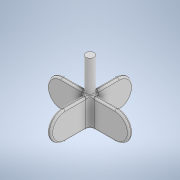
# Autodesk Inventor part: torniquete
Saved by Autodesk Inventor 2022 (Build 260153000, 153)
## iProperties
Created: 2022-11-08
Part Number: torniquete
Material: Generic
Document SubType Name: Modeling
Designer: 3.6b
Density: 1 g/cm^3
Appearance: Default
Author: 3.6b
Autodesk Inventor part; units mm, degrees
ref_plane "YZ Plane" through (0, 0, 0) normal (1, 0, 0) x (0, 1, 0)
ref_plane "XZ Plane" through (0, 0, 0) normal (0, 1, 0) x (-1, 0, 0)
ref_plane "XY Plane" through (0, 0, 0) normal (0, 0, 1) x (1, 0, 0)
sketch "Sketch1" plane through (0, 0, 0) normal (0, 1, 0) x (-1, 0, 0)
  line L0 (33, 2.5) -> (33, -2.5)
  line L1 (-33, -2.5) -> (-33, 2.5)
  line L2 (-33, 2.5) -> (33, -2.5) construction
  line L3 (33, 2.5) -> (-33, -2.5) construction
  line L4 (2.5, 33) -> (-2.5, 33)
  line L5 (-2.5, -33) -> (2.5, -33)
  line L6 (2.5, 33) -> (-2.5, -33) construction
  line L7 (-2.5, 33) -> (2.5, -33) construction
  line L8 (-2.5, 33) -> (-2.5, 2.5)
  line L9 (-2.5, -2.5) -> (-2.5, -33)
  line L10 (2.5, 2.5) -> (2.5, 33)
  line L11 (2.5, -33) -> (2.5, -2.5)
  line L12 (33, -2.5) -> (2.5, -2.5)
  line L13 (-2.5, -2.5) -> (-33, -2.5)
  line L14 (2.5, 2.5) -> (33, 2.5)
  line L15 (-33, 2.5) -> (-2.5, 2.5)
  point P0 (0, 0)
  dimension "d0" = 66
  dimension "d1" = 5
  dimension "d2" = 5
  dimension "d3" = 66
  constraints: 32 end point, 10 parallel, 4 midpoint, 4 perpendicular, 3 horizontal
  measures "d0" distance of L0.end L1.start
  measures "d1" distance of L0.start L0.end
  measures "d2" distance of L5.end L5.start
  measures "d3" distance of L5.start L4.end
extrude "Extrusion1" add sketch "Sketch1" along normal blind 34
sketch "Sketch3" plane through (2.5, 0, 2.5) normal (0, 0, 1) x (1, 0, 0)
  line L0 (30.5, 0) -> (30.5, 34) projected
  line L1 (0, 0) -> (30.5, 0) projected
  arc A0 (30.5, 0) -> (30.5, 34) centre (30.5, 17) ccw
  line L2 (-35.5, 0) -> (-35.5, 34) projected
  arc A1 (-35.5, 34) -> (-35.5, 0) centre (-35.5, 17) ccw
  point P0 (-2.5, 0)
  constraints: 4 end point, 4 point on circle, 2 centre point, 2 midpoint
extrude "Extrusion2" add sketch "Sketch3" against normal blind 5
sketch "Sketch4" plane through (-2.5, 0, -33) normal (-1, 0, 0) x (0, 0, 1)
  line L0 (0, 0) -> (0, 34) projected
  line L1 (0, 34) -> (30.5, 34) projected
  arc A0 (0, 34) -> (0, 0) centre (0, 17) ccw
  line L2 (66, 0) -> (66, 34) projected
  arc A1 (66, 0) -> (66, 34) centre (66, 17) ccw
  point P0 (33, 0)
  constraints: 4 end point, 4 point on circle, 2 centre point, 2 midpoint
extrude "Extrusion3" add sketch "Sketch4" against normal blind 5
sketch "Sketch5" plane through (0, 34, 0) normal (0, 1, 0) x (1, 0, 0)
  circle A0 centre (0, 0) radius 5
  dimension "d10" = 10
  constraints: 1 centre point, 1 coincident
  measures "d10" diameter of A0
extrude "Extrusion4" add sketch "Sketch5" along normal blind 40
fillet "Fillet1" radius 5 1 edges at (-2.5, 17, 2.5)
fillet "Fillet2" radius 5 3 edges at (2.5, 17, 2.5) (2.5, 17, -2.5) (-2.5, 17, -2.5)
fillet "Fillet3" radius 2 1 edges at (-5, 34, 0)
fillet "Fillet4" radius 2 40 edges at (3.9668, 34.5653, 3.9622) (2.5254, 34, 6.9968) (2.5, 34, 20.25) (2.5, 17, 50) (2.5, 0, 20.25) (3.9645, 0, 3.9645) (20.25, 0, 2.5) (50, 17, 2.5) (20.25, 34, 2.5) (6.9968, 34, 2.5254) (6.9968, 34, -2.5254) (20.25, 34, -2.5) (50, 17, -2.5) (20.25, 0, -2.5) (3.9645, 0, -3.9645) (2.5, 0, -20.25) (2.5, 17, -50) (2.5, 34, -20.25) (2.5254, 34, -6.9968) (3.9622, 34.5653, -3.9668) (-2.5254, 34, -6.9968) (-2.5, 34, -20.25) (-2.5, 17, -50) (-2.5, 0, -20.25) (-3.9645, 0, -3.9645) (-20.25, 0, -2.5) (-50, 17, -2.5) (-20.25, 34, -2.5) (-6.9968, 34, -2.5254) (-3.9668, 34.5653, -3.9622) (-6.9968, 34, 2.5254) (-20.25, 34, 2.5) (-50, 17, 2.5) (-20.25, 0, 2.5) (-3.9645, 0, 3.9645) (-2.5, 0, 20.25) (-2.5, 17, 50) (-2.5, 34, 20.25) (-2.5254, 34, 6.9968) (-3.9622, 34.5653, 3.9668)
body "Solid1"
